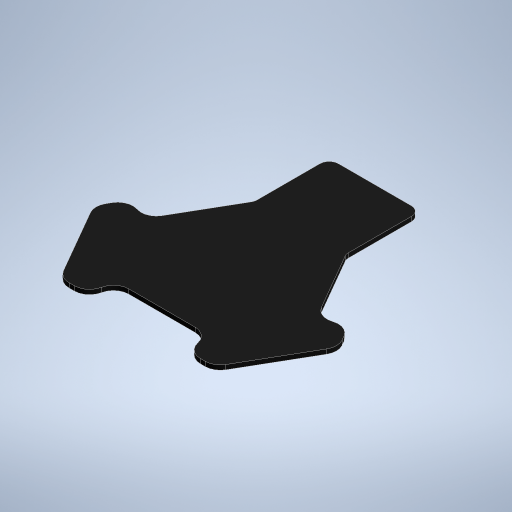
# Autodesk Inventor part: CORE_outline
Saved by Autodesk Inventor 2024.1 (Build 281209000, 209)
## iProperties
Created: 2025-02-03
Part Number: CORE_outline
Material: 一般
Document SubType Name: モデリング
Designer: hibik
Density: 1 g/cm^3
Appearance: 既定
Author: hibik
Autodesk Inventor part; units mm, degrees
ref_plane "YZ Plane" through (0, 0, 0) normal (1, 0, 0) x (0, 1, 0)
ref_plane "XZ Plane" through (0, 0, 0) normal (0, 1, 0) x (-1, 0, 0)
ref_plane "XY Plane" through (0, 0, 0) normal (0, 0, 1) x (1, 0, 0)
sketch "スケッチ1" plane through (0, 0, 0) normal (0, 1, 0) x (-1, 0, 0)
  line L0 (75, 0) -> (105, -51.9615)
  line L1 (-75, 0) -> (-105, -51.9615)
  line L2 (0, -218.2384) -> (0, 36.3731)
  line L3 (147, 0) -> (-147, 0)
  line L4 (37.5, -27) -> (-37.5, -27)
  line L5 (105, -51.9615) -> (30, -181.8653)
  line L6 (30, -181.8653) -> (-30, -181.8653)
  line L7 (-30, -181.8653) -> (-105, -51.9615)
  line L8 (75, 0) -> (-75, 0)
  line L9 (-25.3673, -135.8894) -> (-62.8673, -70.9375)
  line L10 (25.3673, -135.8894) -> (62.8673, -70.9375)
  line L11 (-37.5, -27) -> (-27.5, -27)
  line L12 (-27.5, -27) -> (-27.5, -39)
  line L13 (-27.5, -39) -> (-37.5, -39)
  line L14 (-37.5, -39) -> (-37.5, -27)
  line L15 (37.5, -27) -> (27.5, -27)
  line L16 (27.5, -27) -> (27.5, -39)
  line L17 (27.5, -39) -> (37.5, -39)
  line L18 (37.5, -39) -> (37.5, -27)
  line L19 (0, -77.9423) -> (44.1173, -103.4134) construction
  line L20 (0, -77.9423) -> (-44.1173, -103.4134) construction
  line L21 (-44.1173, -103.4134) -> (-67.5, -116.9134) construction
  line L22 (-57.8673, -79.5977) -> (-47.475, -73.5977)
  line L23 (-52.475, -64.9375) -> (-62.8673, -70.9375)
  line L24 (-62.8673, -70.9375) -> (-57.8673, -79.5977)
  line L25 (-47.475, -73.5977) -> (-52.475, -64.9375)
  line L26 (-25.3673, -135.8894) -> (-30.3673, -127.2291)
  line L27 (-19.975, -121.2291) -> (-14.975, -129.8894)
  line L28 (-14.975, -129.8894) -> (-25.3673, -135.8894)
  line L29 (-30.3673, -127.2291) -> (-19.975, -121.2291)
  line L30 (30.3673, -127.2291) -> (19.975, -121.2291)
  line L31 (14.975, -129.8894) -> (25.3673, -135.8894)
  line L32 (25.3673, -135.8894) -> (30.3673, -127.2291)
  line L33 (19.975, -121.2291) -> (14.975, -129.8894)
  line L34 (62.8673, -70.9375) -> (57.8673, -79.5977)
  line L35 (47.475, -73.5977) -> (52.475, -64.9375)
  line L36 (52.475, -64.9375) -> (62.8673, -70.9375)
  line L37 (57.8673, -79.5977) -> (47.475, -73.5977)
  line L38 (62.8673, -70.9375) -> (37.5, -27)
  line L39 (-37.5, -27) -> (-62.8673, -70.9375)
  line L40 (-25.3673, -135.8894) -> (25.3673, -135.8894)
  line L41 (-25.3673, -135.8894) -> (-25.3673, -181.8653)
  line L42 (25.3673, -135.8894) -> (25.3673, -181.8653)
  line L43 (-25.3673, -135.8894) -> (-48.75, -149.3894)
  line L44 (25.3673, -135.8894) -> (48.75, -149.3894)
  point P0 (0, 0)
  point P1 (0, 0)
  point P2 (0, -27)
  dimension "d1" = 150
  dimension "d2" = 60
  dimension "d3" = 60
  dimension "d4" = 27
  dimension "d5" = 75
  dimension "d6" = 60
  dimension "d7" = 27
  dimension "d8" = 10
  dimension "d9" = 12
  dimension "d10" = 10
  dimension "d11" = 12
  dimension "d14" = 360
  measures "d1" distance of L1.start L0.start
  measures "d2" angle of L3 L0
  measures "d3" angle of L1 L3
  measures "d4" distance between parallel lines of L3 L4
  measures "d5" distance of L4.start L4.end
  measures "d6" distance of L5.end L6.end
  measures "d7" distance between parallel lines of L7 L9
  measures "d8" distance of L12.end L13.end
  measures "d9" distance of L11.end L12.end
  measures "d10" distance of L17.end L16.end
  measures "d11" distance of L16.end L15.end
extrude "プレート1" add sketch "スケッチ1" along normal blind 1.5 contours L5 L6 L42 L44 | L4 L16 L17 L18 L38 L36 L35 L37 L10 L30 L33 L31 L40 L2 | L2 L40 L28 L27 L29 L9 L22 L25 L23 L39 L14 L13 L12 L4 | L31 L33 L30 L10 | L42 L6 L2 L40 | L2 L6 L41 L40 | L4 L18 L17 L16 | L12 L13 L14 L4 | L9 L29 L27 L28 | L41 L6 L7 L43 | L37 L35 L36 L10 | L23 L25 L22 L9
sketch "スケッチ2" plane through (0, 0, 0) normal (0, -1, 0) x (1, 0, 0)
  line L0 (23.3798, -38.55) -> (-23.3798, -38.55) projected
  line L1 (8.2, -46.6) -> (-8.2, -46.6) projected
  arc A0 (-21.1, -27) -> (-23.3798, -38.55) centre (-21.1, -33) ccw projected
  line L2 (-27.5, -27) -> (-27.5, -39) projected
  line L3 (27.5, -39) -> (27.5, -27) projected
  line L4 (-27.5, -39) -> (-27.5, -40.55)
  line L5 (-27.5, -40.55) -> (-10.2, -40.55)
  line L6 (-10.2, -40.55) -> (-10.2, -48.6)
  line L7 (-10.2, -48.6) -> (10.2, -48.6)
  line L8 (10.2, -48.6) -> (10.2, -40.55)
  line L9 (10.2, -40.55) -> (27.5, -40.55)
  line L10 (27.5, -40.55) -> (27.5, -39)
  line L11 (-37.5, -27) -> (-27.5, -27) projected
  line L12 (-37.5, -27) -> (37.5, -27) projected
  line L13 (-20.3112, -101.4469) -> (-30.5112, -83.78)
  line L14 (-27.2827, -105.4719) -> (-20.3112, -101.4469)
  line L15 (-18.6327, -120.4541) -> (-27.2827, -105.4719)
  line L16 (-19.975, -121.2291) -> (-18.6327, -120.4541)
  line L17 (-37.4827, -87.805) -> (-46.1327, -72.8227)
  line L18 (-46.1327, -72.8227) -> (-47.475, -73.5977)
  line L19 (-30.5112, -83.78) -> (-37.4827, -87.805)
  line L20 (30.5112, -83.78) -> (20.3112, -101.4469)
  line L21 (37.4827, -87.805) -> (30.5112, -83.78)
  line L22 (46.1327, -72.8227) -> (37.4827, -87.805)
  line L23 (47.475, -73.5977) -> (46.1327, -72.8227)
  line L24 (27.2827, -105.4719) -> (18.6327, -120.4541)
  line L25 (18.6327, -120.4541) -> (19.975, -121.2291)
  line L26 (20.3112, -101.4469) -> (27.2827, -105.4719)
  line L27 (-47.475, -73.5977) -> (-57.8673, -79.5977)
  line L28 (-57.8673, -79.5977) -> (-30.3673, -127.2291)
  line L29 (-30.3673, -127.2291) -> (-19.975, -121.2291)
  line L30 (19.975, -121.2291) -> (30.3673, -127.2291)
  line L31 (30.3673, -127.2291) -> (57.8673, -79.5977)
  line L32 (57.8673, -79.5977) -> (47.475, -73.5977)
  point P0 (0, 0)
  point P1 (0, -77.9423)
  point P2 (-23.0432, -100.7148)
  point P3 (-33.5673, -121.6866)
  point P4 (-22.4248, -117.8859)
  point P5 (-25.3673, -135.8894)
  point P6 (-28.3712, -118.6866)
  point P7 (-31.2432, -86.512)
  point P8 (-45.8046, -77.3909)
  point P9 (-62.8673, -70.9375)
  point P10 (31.2432, -86.512)
  point P11 (54.6673, -85.1403)
  point P12 (45.8046, -77.3909)
  point P13 (62.8673, -70.9375)
  point P14 (49.4712, -82.1403)
  point P15 (23.0432, -100.7148)
  point P16 (22.4248, -117.8859)
  point P17 (25.3673, -135.8894)
  dimension "d17" = 2
  dimension "d18" = 2
  dimension "d19" = 2
  dimension "d20" = 2
  dimension "d26" = 360
  constraints: 54 end point, 9 perpendicular, 1 collinear, 1 horizontal, 1 vertical, 76 other
  measures "d17" distance between parallel lines of L0 L5
  measures "d18" distance from line of L1.end L6
  measures "d19" distance from line of L8 L1.start
  measures "d20" distance between parallel lines of L7 L1
extrude "切り取り1" cut sketch "スケッチ2" against normal blind 1.5
fillet "フィレット1" radius 1.5 18 edges at (-10.2, 0.75, -48.6) (-10.2, 0.75, -40.55) (-27.5, 0.75, -40.55) (10.2, 0.75, -48.6) (10.2, 0.75, -40.55) (27.5, 0.75, -40.55) (-30.5112, 0.75, -83.78) (-46.1327, 0.75, -72.8227) (-20.3112, 0.75, -101.4469) (-27.2827, 0.75, -105.4719) (-37.4827, 0.75, -87.805) (-18.6327, 0.75, -120.4541) (20.3112, 0.75, -101.4469) (27.2827, 0.75, -105.4719) (18.6327, 0.75, -120.4541) (30.5112, 0.75, -83.78) (37.4827, 0.75, -87.805) (46.1327, 0.75, -72.8227)
sketch "スケッチ3" plane through (0, 0, 0) normal (0, -1, 0) x (1, 0, 0)
  circle A0 centre (40.9875, -45.0405) radius 1.6 projected
  circle A1 centre (48.9875, -58.8969) radius 1.6 projected
  circle A2 centre (8, -129.8894) radius 1.6 projected
  circle A3 centre (-8, -129.8894) radius 1.6 projected
  circle A4 centre (-48.9875, -58.8969) radius 1.6 projected
  circle A5 centre (-40.9875, -45.0405) radius 1.6 projected
  point P0 (0, 0)
extrude "切り取り2" cut sketch "スケッチ3" against normal blind 1.5
sketch "スケッチ4" plane through (0, 0, 0) normal (0, -1, 0) x (1, 0, 0)
  circle A0 centre (10, -176.8653) radius 1.35 projected
  circle A1 centre (21.2333, -145.0496) radius 1.6 projected
  circle A2 centre (10, -143.8894) radius 1.6 projected
  line L0 (52.75, -142.4612) -> (30, -181.8653) projected
  line L1 (52.75, -142.4612) -> (33.6974, -131.4612) projected
  line L2 (33.6974, -131.4612) -> (27.1974, -142.7195) projected
  line L3 (27.1974, -142.7195) -> (20.5635, -138.8894) projected
  line L4 (20.5635, -138.8894) -> (5, -138.8894) projected
  line L5 (5, -138.8894) -> (5, -181.8653) projected
  line L6 (30, -181.8653) -> (5, -181.8653) projected
  circle A3 centre (-10, -176.8653) radius 1.35 projected
  circle A4 centre (-21.2333, -145.0496) radius 1.6 projected
  circle A5 centre (-10, -143.8894) radius 1.6 projected
  line L7 (-12.9295, -171.4323) -> (-35.4295, -132.4612) projected
  line L8 (-30.25, -181.4323) -> (-12.9295, -171.4323) projected
  line L9 (-30, -181.8653) -> (-30.25, -181.4323) projected
  line L10 (-30, -181.8653) -> (-5, -181.8653) projected
  line L11 (-5, -181.8653) -> (-5, -138.8894) projected
  line L12 (-5, -138.8894) -> (-20.5635, -138.8894) projected
  line L13 (-20.5635, -138.8894) -> (-27.1974, -142.7195) projected
  line L14 (-33.6974, -131.4612) -> (-27.1974, -142.7195) projected
  line L15 (-35.4295, -132.4612) -> (-33.6974, -131.4612) projected
  point P0 (0, 0)
extrude "切り取り3" cut sketch "スケッチ4" against normal blind 1.5 contours A0 | A1 | A2 | A3 | A4 | A5
sketch "スケッチ5" plane through (0, 1.5, 0) normal (0, 1, 0) x (1, 0, 0)
  line L0 (-19.975, 121.2291) -> (19.975, 121.2291) projected
  line L1 (47.475, 73.5977) -> (27.5, 39) projected
  line L2 (-47.475, 73.5977) -> (-27.5, 39) projected
  point P0 (0, 0)
sketch "スケッチ6" plane through (0, 1.5, 0) normal (0, 1, 0) x (1, 0, 0)
  line L0 (-26.0855, 44.55) -> (-41.9613, 72.0477)
  line L1 (-41.9613, 72.0477) -> (-36.0186, 82.3409)
  line L2 (-36.0186, 82.3409) -> (-29.0471, 78.3159)
  line L3 (-29.0471, 78.3159) -> (-14.8471, 102.911)
  line L4 (-14.8471, 102.911) -> (-21.8186, 106.936)
  line L5 (-21.8186, 106.936) -> (-15.8758, 117.2291)
  line L6 (-15.8758, 117.2291) -> (15.8758, 117.2291)
  line L7 (15.8758, 117.2291) -> (21.8186, 106.936)
  line L8 (21.8186, 106.936) -> (14.8471, 102.911)
  line L9 (14.8471, 102.911) -> (29.0471, 78.3159)
  line L10 (29.0471, 78.3159) -> (36.0186, 82.3409)
  line L11 (36.0186, 82.3409) -> (41.9613, 72.0477)
  line L12 (41.9613, 72.0477) -> (26.0855, 44.55)
  line L13 (26.0855, 44.55) -> (14.2, 44.55)
  line L14 (14.2, 44.55) -> (14.2, 52.6)
  line L15 (14.2, 52.6) -> (-14.2, 52.6)
  line L16 (-14.2, 52.6) -> (-14.2, 44.55)
  line L17 (-14.2, 44.55) -> (-26.0855, 44.55)
  line L18 (-47.475, 73.5977) -> (-27.5, 39) projected
  line L19 (-38.2327, 86.5059) -> (-45.3827, 74.1218) projected
  line L20 (-31.8102, 84.53) -> (-36.1836, 87.055) projected
  line L21 (-21.0612, 100.1479) -> (-29.7612, 85.079) projected
  line L22 (-25.9836, 104.7219) -> (-21.6102, 102.1969) projected
  line L23 (-19.3827, 119.1551) -> (-26.5327, 106.7709) projected
  line L24 (-19.975, 121.2291) -> (19.975, 121.2291) projected
  line L25 (47.475, 73.5977) -> (27.5, 39) projected
  line L26 (26.5327, 106.7709) -> (19.3827, 119.1551) projected
  line L27 (21.6102, 102.1969) -> (25.9836, 104.7219) projected
  line L28 (29.7612, 85.079) -> (21.0612, 100.1479) projected
  line L29 (36.1836, 87.055) -> (31.8102, 84.53) projected
  line L30 (45.3827, 74.1218) -> (38.2327, 86.5059) projected
  line L31 (11.7, 40.55) -> (26, 40.55) projected
  line L32 (10.2, 47.1) -> (10.2, 42.05) projected
  line L33 (-8.7, 48.6) -> (8.7, 48.6) projected
  line L34 (-10.2, 42.05) -> (-10.2, 47.1) projected
  line L35 (-26, 40.55) -> (-11.7, 40.55) projected
  line L36 (0, 48.6) -> (0, 121.2291)
  line L37 (-25.4112, 92.6134) -> (-31.0836, 95.8884) construction
  point P0 (0, 0)
  dimension "d32" = 4
  dimension "d33" = 4
  dimension "d34" = 4
  dimension "d35" = 4
  dimension "d36" = 4
  dimension "d37" = 4
  dimension "d38" = 4
  dimension "d39" = 4
  dimension "d40" = 4
  constraints: 40 end point, 22 parallel, 3 midpoint, 3 perpendicular, 1 horizontal, 9 other
  measures "d32" distance between parallel lines of L19 L1
  measures "d33" distance between parallel lines of L18 L0
  measures "d34" distance between parallel lines of L21 L3
  measures "d35" distance from line of L20.start L2
  measures "d36" distance between parallel lines of L23 L5
  measures "d37" distance between parallel lines of L24 L6
  measures "d38" distance between parallel lines of L33 L15
  measures "d39" distance from line of L34.end L16
  measures "d40" distance between parallel lines of L35 L17
extrude "切り取り4" cut sketch "スケッチ6" against normal blind 1.5
fillet "フィレット2" radius 5 9 edges at (-14.2, 0.75, -44.55) (-26.0855, 0.75, -44.55) (-41.9613, 0.75, -72.0477) (-36.0186, 0.75, -82.3409) (-21.8186, 0.75, -106.936) (-15.8758, 0.75, -117.2291) (-14.2, 0.75, -52.6) (-29.0471, 0.75, -78.3159) (-14.8471, 0.75, -102.911)
mirror "ミラー1" about plane through (0, 0, 0) normal (1, 0, 0) of "フィレット2"
sketch "スケッチ7" plane through (0, 1.5, 0) normal (0, 1, 0) x (1, 0, 0)
  arc A0 (18.2848, 105.0066) -> (17.2511, 98.7471) centre (21.5812, 101.2471) ccw projected
  line L0 (17.2511, 98.7471) -> (26.643, 82.4797) projected
  arc A1 (26.643, 82.4797) -> (32.5808, 80.2452) centre (30.9732, 84.9797) ccw projected
  arc A2 (38.5186, 78.0107) -> (32.5808, 80.2452) centre (34.1884, 75.5107) ccw projected
  line L1 (38.5186, 78.0107) -> (40.5179, 74.5477) projected
  arc A3 (40.5179, 69.5477) -> (40.5179, 74.5477) centre (36.1878, 72.0477) ccw projected
  line L2 (40.5179, 69.5477) -> (27.5289, 47.05) projected
  arc A4 (23.1987, 44.55) -> (27.5289, 47.05) centre (23.1987, 49.55) ccw projected
  line L3 (23.1987, 44.55) -> (19.2, 44.55) projected
  arc A5 (14.296, 48.575) -> (19.2, 44.55) centre (19.2, 49.55) ccw projected
  arc A6 (14.296, 48.575) -> (9.392, 52.6) centre (9.392, 47.6) ccw projected
  line L4 (9.392, 52.6) -> (-9.392, 52.6) projected
  arc A7 (-9.392, 52.6) -> (-14.296, 48.575) centre (-9.392, 47.6) ccw projected
  arc A8 (-19.2, 44.55) -> (-14.296, 48.575) centre (-19.2, 49.55) ccw projected
  line L5 (-19.2, 44.55) -> (-23.1987, 44.55) projected
  arc A9 (-27.5289, 47.05) -> (-23.1987, 44.55) centre (-23.1987, 49.55) ccw projected
  line L6 (-27.5289, 47.05) -> (-40.5179, 69.5477) projected
  arc A10 (-40.5179, 74.5477) -> (-40.5179, 69.5477) centre (-36.1878, 72.0477) ccw projected
  line L7 (-40.5179, 74.5477) -> (-38.5186, 78.0107) projected
  arc A11 (-32.5808, 80.2452) -> (-38.5186, 78.0107) centre (-34.1884, 75.5107) ccw projected
  arc A12 (-32.5808, 80.2452) -> (-26.643, 82.4797) centre (-30.9732, 84.9797) ccw projected
  line L8 (-26.643, 82.4797) -> (-17.2511, 98.7471) projected
  arc A13 (-17.2511, 98.7471) -> (-18.2848, 105.0066) centre (-21.5812, 101.2471) ccw projected
  arc A14 (-19.3186, 111.2661) -> (-18.2848, 105.0066) centre (-14.9884, 108.7661) ccw projected
  line L9 (-19.3186, 111.2661) -> (-17.3192, 114.7291) projected
  arc A15 (-12.9891, 117.2291) -> (-17.3192, 114.7291) centre (-12.9891, 112.2291) ccw projected
  line L10 (-12.9891, 117.2291) -> (12.9891, 117.2291) projected
  arc A16 (17.3192, 114.7291) -> (12.9891, 117.2291) centre (12.9891, 112.2291) ccw projected
  line L11 (17.3192, 114.7291) -> (19.3186, 111.2661) projected
  arc A17 (18.2848, 105.0066) -> (19.3186, 111.2661) centre (14.9884, 108.7661) ccw projected
  circle A18 centre (21.2333, 145.0496) radius 1.6 projected
  circle A19 centre (-10, 143.8894) radius 1.6 projected
  circle A20 centre (-10, 176.8653) radius 1.35 projected
  circle A21 centre (-21.2333, 145.0496) radius 1.6 projected
  circle A22 centre (10, 176.8653) radius 1.35 projected
  circle A23 centre (10, 143.8894) radius 1.6 projected
  circle A24 centre (-48.9875, 58.8969) radius 1.6 projected
  circle A25 centre (8, 129.8894) radius 1.6 projected
  circle A26 centre (40.9875, 45.0405) radius 1.6 projected
  circle A27 centre (48.9875, 58.8969) radius 1.6 projected
  circle A28 centre (-8, 129.8894) radius 1.6 projected
  circle A29 centre (-40.9875, 45.0405) radius 1.6 projected
  arc A30 (38.2327, 86.5059) -> (36.1836, 87.055) centre (36.9336, 85.7559) ccw projected
  line L12 (36.1836, 87.055) -> (31.8102, 84.53) projected
  arc A31 (29.7612, 85.079) -> (31.8102, 84.53) centre (31.0602, 85.829) ccw projected
  line L13 (29.7612, 85.079) -> (21.0612, 100.1479) projected
  arc A32 (21.6102, 102.1969) -> (21.0612, 100.1479) centre (22.3602, 100.8979) ccw projected
  line L14 (21.6102, 102.1969) -> (25.9836, 104.7219) projected
  arc A33 (25.9836, 104.7219) -> (26.5327, 106.7709) centre (25.2336, 106.0209) ccw projected
  line L15 (26.5327, 106.7709) -> (19.3827, 119.1551) projected
  arc A34 (19.9317, 121.2041) -> (19.3827, 119.1551) centre (20.6817, 119.9051) ccw projected
  line L16 (19.9317, 121.2041) -> (30.3673, 127.2291) projected
  line L17 (25.3673, 135.8894) -> (30.3673, 127.2291) projected
  line L18 (48.75, 149.3894) -> (25.3673, 135.8894) projected
  line L19 (30, 181.8653) -> (48.75, 149.3894) projected
  line L20 (-30, 181.8653) -> (30, 181.8653) projected
  line L21 (-48.75, 149.3894) -> (-30, 181.8653) projected
  line L22 (-25.3673, 135.8894) -> (-48.75, 149.3894) projected
  line L23 (-30.3673, 127.2291) -> (-25.3673, 135.8894) projected
  line L24 (-30.3673, 127.2291) -> (-19.9317, 121.2041) projected
  arc A35 (-19.3827, 119.1551) -> (-19.9317, 121.2041) centre (-20.6817, 119.9051) ccw projected
  line L25 (-19.3827, 119.1551) -> (-26.5327, 106.7709) projected
  arc A36 (-26.5327, 106.7709) -> (-25.9836, 104.7219) centre (-25.2336, 106.0209) ccw projected
  line L26 (-25.9836, 104.7219) -> (-21.6102, 102.1969) projected
  arc A37 (-21.0612, 100.1479) -> (-21.6102, 102.1969) centre (-22.3602, 100.8979) ccw projected
  line L27 (-21.0612, 100.1479) -> (-29.7612, 85.079) projected
  arc A38 (-31.8102, 84.53) -> (-29.7612, 85.079) centre (-31.0602, 85.829) ccw projected
  line L28 (-31.8102, 84.53) -> (-36.1836, 87.055) projected
  arc A39 (-36.1836, 87.055) -> (-38.2327, 86.5059) centre (-36.9336, 85.7559) ccw projected
  line L29 (-38.2327, 86.5059) -> (-45.3827, 74.1218) projected
  arc A40 (-47.4317, 73.5727) -> (-45.3827, 74.1218) centre (-46.6817, 74.8718) ccw projected
  line L30 (-47.4317, 73.5727) -> (-57.8673, 79.5977) projected
  line L31 (-62.8673, 70.9375) -> (-57.8673, 79.5977) projected
  line L32 (-37.5, 27) -> (-62.8673, 70.9375) projected
  line L33 (-27.5, 27) -> (-37.5, 27) projected
  line L34 (-27.5, 27) -> (-27.5, 39.05) projected
  arc A41 (-26, 40.55) -> (-27.5, 39.05) centre (-26, 39.05) ccw projected
  line L35 (-26, 40.55) -> (-11.7, 40.55) projected
  arc A42 (-11.7, 40.55) -> (-10.2, 42.05) centre (-11.7, 42.05) ccw projected
  line L36 (-10.2, 42.05) -> (-10.2, 47.1) projected
  arc A43 (-8.7, 48.6) -> (-10.2, 47.1) centre (-8.7, 47.1) ccw projected
  line L37 (-8.7, 48.6) -> (8.7, 48.6) projected
  arc A44 (10.2, 47.1) -> (8.7, 48.6) centre (8.7, 47.1) ccw projected
  line L38 (10.2, 47.1) -> (10.2, 42.05) projected
  arc A45 (10.2, 42.05) -> (11.7, 40.55) centre (11.7, 42.05) ccw projected
  line L39 (11.7, 40.55) -> (26, 40.55) projected
  arc A46 (27.5, 39.05) -> (26, 40.55) centre (26, 39.05) ccw projected
  line L40 (27.5, 39.05) -> (27.5, 27) projected
  line L41 (37.5, 27) -> (27.5, 27) projected
  line L42 (62.8673, 70.9375) -> (37.5, 27) projected
  line L43 (57.8673, 79.5977) -> (62.8673, 70.9375) projected
  line L44 (57.8673, 79.5977) -> (47.4317, 73.5727) projected
  arc A47 (45.3827, 74.1218) -> (47.4317, 73.5727) centre (46.6817, 74.8718) ccw projected
  line L45 (45.3827, 74.1218) -> (38.2327, 86.5059) projected
  line L46 (25.2195, 46.05) -> (15.796, 46.05)
  line L47 (15.796, 46.05) -> (15.796, 54.1)
  line L48 (15.796, 54.1) -> (-15.796, 54.1)
  line L49 (-15.796, 54.1) -> (-15.796, 46.05)
  line L50 (-15.796, 46.05) -> (-25.2195, 46.05)
  line L51 (-25.2195, 46.05) -> (-40.2293, 72.0477)
  line L52 (-40.2293, 72.0477) -> (-35.5175, 80.2087)
  line L53 (-35.5175, 80.2087) -> (-28.546, 76.1837)
  line L54 (-28.546, 76.1837) -> (-12.75, 103.5432)
  line L55 (-12.75, 103.5432) -> (-19.7215, 107.5682)
  line L56 (-19.7215, 107.5682) -> (-15.0098, 115.7291)
  line L57 (-15.0098, 115.7291) -> (15.0098, 115.7291)
  line L58 (15.0098, 115.7291) -> (19.7215, 107.5682)
  line L59 (19.7215, 107.5682) -> (12.75, 103.5432)
  line L60 (12.75, 103.5432) -> (28.546, 76.1837)
  line L61 (28.546, 76.1837) -> (35.5175, 80.2087)
  line L62 (35.5175, 80.2087) -> (40.2293, 72.0477)
  line L63 (40.2293, 72.0477) -> (25.2195, 46.05)
  line L64 (0, 54.1) -> (0, 115.7291) construction
  line L65 (0, 218.2384) -> (0, -36.3731) construction
  line L66 (40.5179, 69.5477) -> (27.5289, 47.05) projected
  line L67 (20.648, 89.8634) -> (0, 77.9423) construction
  line L68 (0, 54.1) -> (0, 77.9423) construction
  line L69 (17.3192, 114.7291) -> (19.3186, 111.2661) projected
  point P0 (0, 0)
  dimension "d44" = 1.5
  dimension "d45" = 1.5
  dimension "d46" = 1.5
  dimension "d47" = 1.5
  dimension "d48" = 1.5
  dimension "d49" = 1.5
  dimension "d50" = 1.5
  dimension "d51" = 1.5
  constraints: 42 end point, 7 perpendicular, 5 parallel, 4 midpoint, 2 vertical, 1 collinear, 1 equal length, 1 horizontal, 1 point on line, 8 other
  measures "d44" distance between parallel lines of L3 L46
  measures "d45" distance between parallel lines of L66 L63
  measures "d46" distance between parallel lines of L1 L62
  measures "d47" distance between parallel lines of L0 L60
  measures "d48" distance from line of A1.end L61
  measures "d49" distance between parallel lines of L4 L48
  measures "d50" distance from line of A5.start L47
  measures "d51" distance between parallel lines of L10 L57
extrude "押し出し1" cut sketch "スケッチ7" against normal through all contours A0 L0 A1 A2 L1 A3 L2 A4 L3 A5 A6 L4 A7 A8 L5 A9 L6 A10 L7 A11 A12 L8 A13 A14 L9 A15 L10 A16 L11 A17 | L45 A47 L44 L43 L42 L41 L40 A46 L39 A45 L38 A44 L37 A43 L36 A42 L35 A41 L34 L33 L32 L31 L30 A40 L29 A39 L28 A38 L27 A37 L26 A36 L25 A35 L24 L23 L22 L21 L20 L19 L18 L17 L16 A34 L15 A33 L14 A32 L13 A31 L12 A30 | L46 L47 L48 L49 L50 L51 L52 L53 L54 L55 L56 L57 L58 L59 L60 L61 L62 L63
extrude "押し出し2" add sketch "スケッチ7" along normal blind 1.5 contours L46 L47 L48 L49 L50 L51 L52 L53 L54 L55 L56 L57 L58 L59 L60 L61 L62 L63
sketch "スケッチ8" plane through (0, 3, 0) normal (0, 1, 0) x (1, 0, 0)
  line L0 (15, 59.1) -> (-15, 59.1)
  line L1 (-15, 59.1) -> (-15, 124.1)
  line L2 (-15, 124.1) -> (15, 124.1)
  line L3 (15, 124.1) -> (15, 59.1)
  line L4 (-15.796, 54.1) -> (15.796, 54.1) projected
  line L5 (15.0098, 115.7291) -> (-15.0098, 115.7291) projected
  point P0 (0, 0)
  point P1 (0, 59.1)
  point P2 (0, 54.1)
  point P3 (-15, 115.7291)
  point P4 (15, 115.7291)
  dimension "d56" = 65
  dimension "d57" = 30
  dimension "d58" = 5
  constraints: 8 end point, 2 midpoint, 2 parallel, 1 horizontal, 1 perpendicular, 1 vertical alignment
  measures "d56" distance of L0.end L1.end
  measures "d57" distance of L0.start L0.end
  measures "d58" distance between parallel lines of L4 L0
extrude "押し出し3" add sketch "スケッチ8" against normal up to surface (1.5 mm away) contours L5 L1 L2 L3
fillet "フィレット3" radius 3 4 edges at (15, 2.25, -124.1) (-15, 2.25, -124.1) (-15.0098, 2.25, -115.7291) (15.0098, 2.25, -115.7291)
fillet "フィレット4" radius 5 16 edges at (19.7215, 2.25, -107.5682) (12.75, 2.25, -103.5432) (28.546, 2.25, -76.1837) (35.5175, 2.25, -80.2087) (40.2293, 2.25, -72.0477) (25.2195, 2.25, -46.05) (15.796, 2.25, -46.05) (15.796, 2.25, -54.1) (-15.796, 2.25, -54.1) (-15.796, 2.25, -46.05) (-25.2195, 2.25, -46.05) (-40.2293, 2.25, -72.0477) (-35.5175, 2.25, -80.2087) (-28.546, 2.25, -76.1837) (-12.75, 2.25, -103.5432) (-19.7215, 2.25, -107.5682)
sketch "スケッチ9" plane through (0, 3, 0) normal (0, 1, 0) x (1, 0, 0)
  line L0 (26.046, 80.5138) -> (15.154, 99.3793) projected
  line L1 (-15.25, 99.213) -> (-26.142, 80.3476) projected
  line L2 (-15, 121.1) -> (-15, 115.7291) projected
  line L3 (15, 115.7291) -> (15, 121.1) projected
  line L4 (15, 115.7291) -> (15, 104.0911)
  line L5 (-15, 115.7291) -> (-15, 103.7185)
  arc A0 (16.1878, 105.6388) -> (15.154, 99.3793) centre (19.4842, 101.8793) ccw projected
  arc A1 (-15.25, 99.213) -> (-16.2838, 105.4725) centre (-19.5802, 101.713) ccw projected
  arc A2 (-17.3175, 111.732) -> (-16.2838, 105.4725) centre (-12.9874, 109.232) ccw projected
  line L6 (-15.1201, 115.5381) -> (-17.3175, 111.732) projected
  line L7 (17.2215, 111.8983) -> (15.1201, 115.5381) projected
  arc A3 (16.1878, 105.6388) -> (17.2215, 111.8983) centre (12.8914, 109.3983) ccw projected
  arc A4 (15.1201, 115.5381) -> (15, 115.7291) centre (12.522, 114.0381) ccw projected
  arc A5 (-15, 115.7291) -> (-15.1201, 115.5381) centre (-12.522, 114.0381) ccw projected
  line L8 (-15, 103.7185) -> (-15, 99.6461)
  line L9 (15, 104.0911) -> (15, 99.6461)
  point P0 (0, 0)
  point P1 (-15, 99.7075)
  point P2 (15, 99.6675)
  constraints: 8 end point, 2 collinear, 2 point on circle, 2 point on line, 2 vertical
extrude "押し出し4" cut sketch "スケッチ9" against normal through all contours A4 L7 A3 A0 L4 | L5 A1 A2 L6 A5
extrude "押し出し5" add sketch "スケッチ9" against normal up to surface (1.5 mm away) contours L9 A0 | A1 L8
fillet "フィレット5" radius 3 2 edges at (-15, 2.25, -99.7075) (15, 2.25, -99.6675)
equation "\"d3\" = d2"
equation "\"d7\" = d4"
equation "\"d19\" = d18"
equation "\"d21\" = Thickness"
equation "\"d28\" = Thickness"
equation "\"d30\" = Thickness"
equation "\"d33\" = d32"
equation "\"d34\" = d32"
equation "\"d35\" = d32"
equation "\"d36\" = d32"
equation "\"d37\" = d32"
equation "\"d38\" = d32"
equation "\"d39\" = d32"
equation "\"d40\" = d32"
equation "\"d41\" = Thickness"
equation "\"d45\" = d44"
equation "\"d46\" = d44"
equation "\"d47\" = d44"
equation "\"d48\" = d44"
equation "\"d49\" = d44"
equation "\"d50\" = d44"
equation "\"d51\" = d44"
equation "\"d16\" = Thickness"
equation "\"BendRadius\" = Thickness"
equation "\"BendReliefWidth\" = Thickness"
equation "\"BendReliefDepth\" = 0.5 * Thickness"
equation "\"CornerReliefSize\" = 4 * Thickness"
equation "\"MinimumRemnant\" = 2 * Thickness"
equation "\"TransitionRadius\" = BendRadius"
equation "\"JacobiRadiusSize\" = BendRadius"
equation "\"GapSize\" = Thickness"
equation "\"Thickness\" = 1.5"
